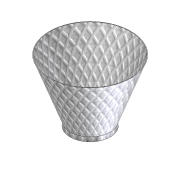
# Autodesk Inventor part: GE-12014
Saved by Autodesk Inventor 2012 (Build 160160000, 160)
## iProperties
Created: 2011-05-26
Part Number: GE-12014
Document SubType Name: Modeling
Designer: dfoster
Density: 1 g/cm^3
Description: Basketball Net
Material: Default
Title: Basketball Net
Author: dfoster
Autodesk Inventor part; units mm, degrees
ref_plane "YZ Plane" through (0, 0, 0) normal (1, 0, 0) x (0, 1, 0)
ref_plane "XZ Plane" through (0, 0, 0) normal (0, 1, 0) x (-1, 0, 0)
ref_plane "XY Plane" through (0, 0, 0) normal (0, 0, 1) x (1, 0, 0)
sketch "Sketch1" plane through (0, 0, 0) normal (0, 0, 1) x (1, 0, 0)
  line L0 (-239.9154, 0) -> (-236.5375, 0)
  line L1 (-236.5375, 0) -> (-114.3, -336.55)
  line L2 (-114.3, -336.55) -> (-117.6779, -336.55)
  line L3 (-117.6779, -336.55) -> (-239.9154, 0)
  line L4 (0, 0) -> (0, -62.0515)
  line L5 (-114.3, -336.55) -> (-114.3, -361.95)
  line L6 (-114.3, -361.95) -> (-117.6779, -361.95)
  line L7 (-117.6779, -361.95) -> (-117.6779, -336.55)
  dimension "d0" = 361.95
  dimension "d1" = 25.4
  dimension "d2" = 0
  dimension "d3" = 236.5375
  dimension "d4" = 3.175
  dimension "d5" = 114.3
  constraints: 16 end point, 4 parallel, 2 perpendicular, 1 horizontal
  measures "d0" distance from line of L4.start L6
  measures "d1" distance of L6.end L2.end
  measures "d2" distance from line of L4.start L0
  measures "d3" distance from line of L0.end L4
  measures "d4" distance between parallel lines of L1 L3
  measures "d5" distance between parallel lines of L5 L4
revolve "Revolution1" add sketch "Sketch1" angle 360 about axis through (0, 0, 0) along (0, -1, 0)
body "Solid1"
